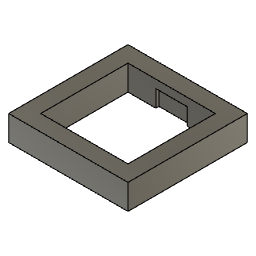
key holder base v1 (Autodesk Fusion 360 design; units mm, degrees)
Autodesk Fusion 360 part; units mm, degrees
sketch "Sketch1" plane through (0, 0, 0) normal (0, 0, 1) x (1, 0, 0)
  line L0 (5.2435, 4.6143) -> (24.2435, 4.6143)
  line L1 (24.2435, 4.6143) -> (24.2435, 23.6143)
  line L2 (24.2435, 23.6143) -> (5.2435, 23.6143)
  line L3 (5.2435, 23.6143) -> (5.2435, 4.6143)
  line L4 (5.2435, 23.6143) -> (24.2435, 4.6143) construction
  line L5 (24.2435, 23.6143) -> (5.2435, 4.6143) construction
  line L6 (5.2435, 4.6143) -> (10.3435, 4.6143) construction
  line L7 (5.2435, 4.6143) -> (7.7935, 4.6143) construction
  line L8 (7.7935, 4.6143) -> (7.7935, 23.6143) construction
  line L9 (7.7935, 7.1643) -> (21.6935, 7.1643)
  line L10 (21.6935, 7.1643) -> (21.6935, 21.0643)
  line L11 (21.6935, 21.0643) -> (7.7935, 21.0643)
  line L12 (7.7935, 21.0643) -> (7.7935, 7.1643)
  dimension "d1" = 19
  dimension "d2" = 19
  dimension "d4" = 2.55
  dimension "d5" = 13.9
  dimension "d6" = 13.9
  constraint horizontal L0
  constraint vertical L1
  constraint horizontal L2
  constraint vertical L3
  constraint perpendicular L3 L6
  constraint perpendicular L3 L7
  constraint coincident L2 L8.end
  constraint perpendicular L2 L8
  constraint horizontal L9
  constraint vertical L10
  constraint horizontal L11
  constraint vertical L12
  constraint coincident L5 L9.start
  constraint coincident L8 L9.start
  measures "d1" distance of L0.start L0.end
  measures "d2" distance of L0.start L2.end
  measures "d4" distance of L0.start L7.end
  measures "d5" distance of L9.start L9.end
  measures "d6" distance of L9.start L11.end
extrude "Extrude1" add sketch "Sketch1" along normal blind 4
sketch "Sketch2" plane through (0, 21.0643, 0) normal (0, -1, 0) x (1, 0, 0)
  line L0 (7.7935, 0) -> (21.6935, 0)
  line L1 (21.6935, 0) -> (21.6935, 4)
  line L2 (21.6935, 4) -> (7.7935, 4)
  line L3 (7.7935, 4) -> (7.7935, 0)
  line L4 (14.7435, 0) -> (17.2435, 0) construction
  line L5 (17.2435, 0) -> (12.2435, 0)
  line L6 (12.2435, 0) -> (12.2435, 2.7)
  line L7 (12.2435, 2.7) -> (17.2435, 2.7)
  line L8 (17.2435, 2.7) -> (17.2435, 0)
  dimension "d9" = 2.5
  dimension "d10" = 5
  dimension "d11" = 2.7
  constraint midpoint L0 L4.start
  constraint parallel L0 L4
  constraint horizontal L5
  constraint vertical L6
  constraint horizontal L7
  constraint vertical L8
  measures "d9" distance of L4.start L4.end
  measures "d10" distance of L4.end L5.end
  measures "d11" distance of L4.end L7.end
extrude "Extrude2" add sketch "Sketch2" along normal blind 0.5 contours L0 L5 L6 L7 L8
extrude "Extrude3" cut 1 faces at (13.9102, 20.5643, 0.9) along direction (0, 1, 0) blind 1
